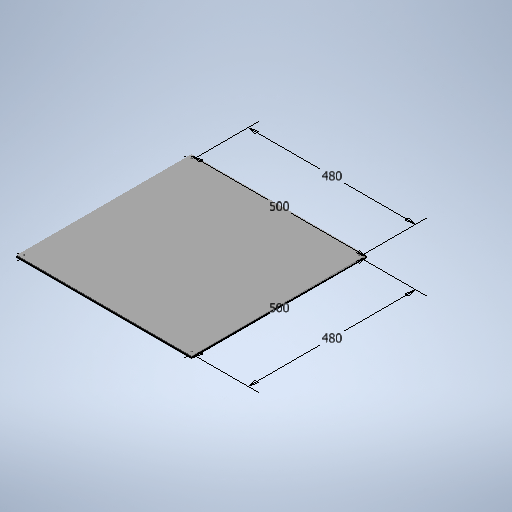
# Autodesk Inventor part: Base
Saved by Autodesk Inventor 2025.4 (Build 294407000, 407)
## iProperties
Created: 2026-07-08
Part Number: Base
Material: Générique
Document SubType Name: Modeling
Designer: louis
Density: 1 g/cm^3
Appearance: Par défaut
Author: louis
Autodesk Inventor part; units mm, degrees
ref_plane "YZ Plane" through (0, 0, 0) normal (1, 0, 0) x (0, 1, 0)
ref_plane "XZ Plane" through (0, 0, 0) normal (0, 1, 0) x (-1, 0, 0)
ref_plane "XY Plane" through (0, 0, 0) normal (0, 0, 1) x (1, 0, 0)
sketch "Sketch2" plane through (0, 0, 0) normal (0, 0, 1) x (1, 0, 0)
  line L0 (-250, -250) -> (250, -250)
  line L1 (250, -250) -> (250, 250)
  line L2 (250, 250) -> (-250, 250)
  line L3 (-250, 250) -> (-250, -250)
  line L4 (-250, -250) -> (250, 250) construction
  line L5 (250, -250) -> (-250, 250) construction
  line L6 (-240, -240) -> (240, -240) construction
  line L7 (240, -240) -> (240, 240) construction
  line L8 (240, 240) -> (-240, 240) construction
  line L9 (-240, 240) -> (-240, -240) construction
  line L10 (-240, -240) -> (240, 240) construction
  line L11 (240, -240) -> (-240, 240) construction
  point P0 (0, 0)
  dimension "d0" = 500
  dimension "d1" = 500
  dimension "d2" = 480
  dimension "d3" = 480
  constraints: 24 end point, 4 coincident, 4 midpoint, 4 parallel, 2 horizontal, 2 perpendicular
  measures "d0" distance of L2.end L1.end
  measures "d1" distance of L1.end L0.end
  measures "d2" distance of L8.end L7.end
  measures "d3" distance of L7.end L6.end
extrude "Extrusion1" add sketch "Sketch2" along normal blind 5
hole "Hole1" at (-240, 240, 0) at (240, 240, 0) at (240, -240, 0) at (-240, -240, 0) direction (0, 0, 1) diameter 5.5 end through all clearance for "Flat Head Machine Screw" size "M5" standard "Ansi Metric M Profile"
fillet "Fillet1" radius 2 4 edges at (250, 250, 2.5) (250, -250, 2.5) (-250, -250, 2.5) (-250, 250, 2.5)
body "Solid1"
